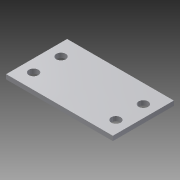
# Autodesk Inventor part: Line trace catch
Saved by Autodesk Inventor 2015 (Build 190159000, 159)
## iProperties
Created: 2015-06-22
Part Number: Line trace catch
Material: アルミニウム 5052 H32
Document SubType Name: Modeling
Designer: kenta
Density: 2.68 g/cm^3
Appearance: サテン
Mass: 2.69263 g
Surface Area: 15.6305 cm^2
Volume: 1.00471 cm^3
Author: kenta
Autodesk Inventor part; units mm, degrees
ref_plane "YZ Plane" through (0, 0, 0) normal (1, 0, 0) x (0, 1, 0)
ref_plane "XZ Plane" through (0, 0, 0) normal (0, 1, 0) x (-1, 0, 0)
ref_plane "XY Plane" through (0, 0, 0) normal (0, 0, 1) x (1, 0, 0)
sketch "スケッチ1" plane through (0, 0, 0) normal (0, 0, 1) x (1, 0, 0)
  line L0 (-17.5, 10) -> (17.5, 10)
  line L1 (17.5, 10) -> (17.5, -10)
  line L2 (17.5, -10) -> (-17.5, -10)
  line L3 (-17.5, -10) -> (-17.5, 10)
  line L4 (-17.5, 10) -> (17.5, -10) construction
  line L5 (17.5, 10) -> (-17.5, -10) construction
  point P0 (0, 0)
  dimension "d0" = 35
  dimension "d1" = 20
  constraints: 12 end point, 2 midpoint, 2 parallel, 1 horizontal, 1 perpendicular
  measures "d0" distance of L1.end L2.end
  measures "d1" distance of L0.end L1.end
extrude "押し出し1" add sketch "スケッチ1" along normal blind 1.5
sketch "スケッチ2" plane through (0, 0, 1.5) normal (0, 0, 1) x (1, 0, 0)
  line L0 (-17.5, -10) -> (-17.5, 10) projected
  line L1 (17.5, -10) -> (-17.5, -10) projected
  point P0 (0, 0)
  point P1 (-13.5, -5)
  point P2 (13.5, -5)
  point P3 (-13.5, 4)
  point P4 (13.5, 4)
  dimension "d4" = 27
  dimension "d5" = 4
  dimension "d6" = 5
  dimension "d15" = 9
  constraints: 2 horizontal alignment, 2 vertical alignment
  measures "d4" distance of point (13.5, -5) point (-13.5, -5)
  measures "d5" distance from line of point (-13.5, -5) L0
  measures "d6" distance from line of point (-13.5, -5) L1
  measures "d15" distance of point (-13.5, -5) point (-13.5, 4)
hole "穴1" at (-13.5, -5, 1.5) at (13.5, -5, 1.5) at (-13.5, 4, 1.5) at (13.5, 4, 1.5) direction (0, 0, -1) diameter 3.1 end through all
